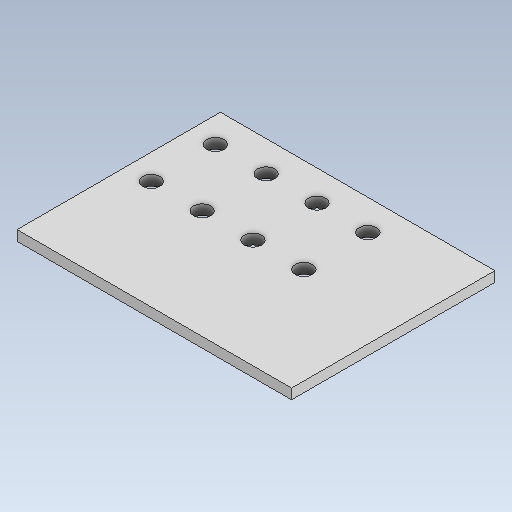
# Autodesk Inventor part: Lift.03.01.00.02
Saved by Autodesk Inventor 2021 (Build 250183000, 183)
## iProperties
Created: 2020-09-20
Part Number: Lift.03.01.00.02
Material: Типовые
Document SubType Name: ЛистМат
Designer: Kostya
Density: 1 g/cm^3
Sheet Metal Rule: По умолчанию_мм
Appearance: По умолчанию
Author: Kostya
Autodesk Inventor part; units mm, degrees
ref_plane "YZ Plane" through (0, 0, 0) normal (1, 0, 0) x (0, 1, 0)
ref_plane "XZ Plane" through (0, 0, 0) normal (0, 1, 0) x (-1, 0, 0)
ref_plane "XY Plane" through (0, 0, 0) normal (0, 0, 1) x (1, 0, 0)
sketch "Эскиз1" plane through (0, 0, 0) normal (0, 1, 0) x (-1, 0, 0)
  line L0 (-135, -100) -> (135, -100)
  line L1 (135, -100) -> (135, 100)
  line L2 (135, 100) -> (-135, 100)
  line L3 (-135, 100) -> (-135, -100)
  line L4 (-135, -100) -> (135, 100) construction
  line L5 (135, -100) -> (-135, 100) construction
  circle A0 centre (110, -70) radius 8.5
  circle A1 centre (110, -7) radius 8.5
  circle A2 centre (60, -7) radius 8.5
  circle A3 centre (60, -70) radius 8.5
  circle A4 centre (10, -7) radius 8.5
  circle A5 centre (10, -70) radius 8.5
  circle A6 centre (-40, -7) radius 8.5
  circle A7 centre (-40, -70) radius 8.5
  point P0 (0, 0)
  dimension "d0" = 270
  dimension "d1" = 200
  dimension "d2" = 30
  dimension "d3" = 63
  dimension "d4" = 95
  dimension "d5" = 50
  dimension "d6" = 50
  dimension "d7" = 50
  dimension "d8" = 17
  measures "d0" distance of L2.end L1.end
  measures "d1" distance of L1.end L0.end
  measures "d2" distance from line of L0 A0.centre
  measures "d3" distance of A1.centre A0.centre
  measures "d4" distance from line of A7.centre L3
  measures "d5" distance of A7.centre A5.centre
  measures "d6" distance of A3.centre A5.centre
  measures "d7" distance of A3.centre A0.centre
  measures "d8" diameter of A0
extrude "Пластина1" add sketch "Эскиз1" along normal blind 10
equation "\"d6\" = d5"
equation "\"d7\" = d6"
equation "\"d9\" = Толщина"
equation "\"Глубина_просечки\" = 0.5 * Толщина"
equation "\"Толщина\" = 10"
